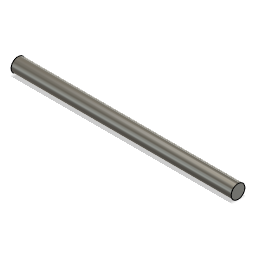
axle v7 (Autodesk Fusion 360 design; units mm, degrees)
Autodesk Fusion 360 part; units mm, degrees
sketch "Sketch1" plane through (0, 0, 0) normal (0, 0, 1) x (1, 0, 0)
sketch "Sketch2" plane through (0, 0, 0) normal (1, 0, 0) x (0, 0, -1)
  circle A0 centre (0, 0) radius 2.5
  dimension "d1" = 5
  constraint coincident A0.centre origin
  measures "d1" diameter of A0
extrude "Extrude1" add sketch "Sketch2" along normal blind 70
extrude "Extrude2" add 1 faces at (70, 0.2321, 0.8863) along direction (1, 0, 0) blind 20
extrude "Extrude3" cut 1 faces at (0, 0.2321, 0.8863) along direction (1, 0, 0) blind 10
extrude "Extrude4" cut 1 faces at (10, 0.2321, 0.8863) along direction (1, 0, 0) blind 10
extrude "Extrude5" add 1 faces at (20, 0.2321, 0.8863) along direction (-1, 0, 0) blind 10
